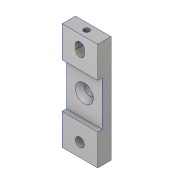
# Autodesk Inventor part: RollerBracket
Saved by Autodesk Inventor 2018 (Build 220112000, 112)
## iProperties
Created: 2020-01-17
Part Number: RollerBracket
Material: Aluminum 6061
Document SubType Name: Modeling
Designer: 22perngrac
Density: 2.7 g/cm^3
Appearance: Aluminum - Flat
Mass: 39.0791 g
Surface Area: 60.9228 cm^2
Volume: 14.4737 cm^3
Author: 22perngrac
Autodesk Inventor part; units mm, degrees
ref_plane "YZ Plane" through (0, 0, 0) normal (1, 0, 0) x (0, 1, 0)
ref_plane "XY Plane" through (0, 0, 0) normal (0, 0, 1) x (1, 0, 0)
sketch "Sketch1" plane through (0, 0, 0) normal (0, 0, 1) x (1, 0, 0)
  line L0 (0, 0) -> (25.4, 0)
  line L1 (25.4, 0) -> (25.4, 76.2)
  line L2 (25.4, 76.2) -> (0, 76.2)
  line L3 (0, 76.2) -> (0, 0)
  dimension "d0" = 76.2
  dimension "d1" = 25.4
  constraints: 8 end point, 2 parallel, 1 horizontal, 1 perpendicular
  measures "d0" distance of L0.end L1.end
  measures "d1" distance of L1.end L2.end
extrude "Extrusion1" add sketch "Sketch1" along normal blind 6.35
sketch "Sketch2" plane through (0, 0, 6.35) normal (0, 0, 1) x (1, 0, 0)
  line L0 (25.4, 76.2) -> (0, 76.2) projected
  line L1 (25.4, 0) -> (25.4, 76.2) projected
  line L2 (0, 76.2) -> (25.4, 76.2)
  line L3 (25.4, 76.2) -> (25.4, 53.975)
  line L4 (25.4, 53.975) -> (0, 53.975)
  line L5 (0, 53.975) -> (0, 76.2)
  line L6 (0, 0) -> (25.4, 0) projected
  dimension "d4" = 22.225
  constraints: 8 end point, 2 parallel, 1 horizontal, 1 perpendicular, 1 point on line
  measures "d4" distance of L4.end L0.end
extrude "Extrusion2" add sketch "Sketch2" along normal blind 3.175
ref_plane "Work Plane1" through (0, 38.1, 0) normal (0, 1, 0) x (-1, 0, 0)
mirror "Mirror1" about plane through (0, 38.1, 0) normal (0, 1, 0) of "Extrusion2"
sketch "Sketch6" plane through (0, 0, 0) normal (0, 0, 1) x (1, 0, 0)
  line L0 (25.4, 76.2) -> (0, 76.2) projected
  line L1 (25.4, 53.975) -> (25.4, 76.2) projected
  line L2 (25.4, 0) -> (0, 0) projected
  line L3 (0, 22.225) -> (25.4, 22.225) projected
  line L4 (25.4, 22.225) -> (25.4, 0) projected
  point P0 (12.7, 9.525)
  dimension "d28" = 12.7
  dimension "d29" = 12.7
  measures "d28" distance from line of point (12.7, 9.525) L3
  measures "d29" distance from line of point (12.7, 9.525) L4
sketch "Sketch7" plane through (0, 0, 6.35) normal (0, 0, 1) x (1, 0, 0)
  line L0 (0, 53.975) -> (25.4, 53.975) projected
  line L1 (0, 53.975) -> (0, 22.225) projected
  line L2 (25.4, 0) -> (25.4, 76.2) projected
  point P0 (0, 0)
  point P1 (12.7, 38.1)
  point P2 (25.4, 38.1)
  dimension "d38" = 12.7
  constraints: 1 horizontal alignment, 1 midpoint
  measures "d38" distance from line of L1 point (12.7, 38.1)
hole "Hole3" at (12.7, 38.1, 6.35) direction (0, 0, -1) diameter 6.7564 end through all countersink diameter 12.8778 countersink angle 82 clearance for "Flat Head Machine Screw (82)" size "1/4" standard "Ansi Unified Screw Threads"
hole "Hole4" at (12.7, 9.525, 0) direction (0, 0, 1) diameter 6.3754 end through all countersink diameter 12.8778 countersink angle 82 clearance for "Flat Head Machine Screw (82)" size "1/4" standard "Ansi Unified Screw Threads"
sketch "Sketch8" plane through (0, 0, 0) normal (0, 0, -1) x (-1, 0, 0)
  line L0 (-12.7, 68.2625) -> (-12.7, 65.0875) construction
  line L1 (-15.8877, 68.2625) -> (-15.8877, 65.0875)
  line L2 (-9.5123, 65.0875) -> (-9.5123, 68.2625)
  arc A0 (-9.5123, 68.2625) -> (-15.8877, 68.2625) centre (-12.7, 68.2625) ccw
  arc A1 (-15.8877, 65.0875) -> (-9.5123, 65.0875) centre (-12.7, 65.0875) ccw
  circle A2 centre (-12.7, 9.525) radius 6.4389 projected
  point P0 (-12.7, 66.675)
  point P1 (-12.7, 66.675)
  dimension "d54" = 3.175
  dimension "d67" = 57.15
  dimension "d68" = 6.3754
  constraints: 8 end point, 4 point on circle, 4 tangent, 2 centre point, 2 coincident, 1 midpoint, 1 parallel, 1 vertical
  measures "d54" distance of L1.start L1.end
  measures "d67" distance of A2.centre point (-12.7, 66.675)
  measures "d68" diameter of A0
extrude "Extrusion3" cut sketch "Sketch8" against normal through all contours A0 L2 A1 L1
sketch "Sketch10" plane through (0, 76.2, 0) normal (0, 1, 0) x (1, 0, 0)
  line L0 (0, 0) -> (0, -9.525) projected
  line L1 (25.4, 0) -> (0, 0) projected
  point P0 (12.7, -4.7625)
  point P1 (0, -4.7625)
  point P2 (12.7, 0)
  constraints: 2 midpoint, 1 horizontal alignment, 1 vertical alignment
hole "Hole5" at (12.7, 76.2, 4.7625) direction (0, -1, 0) diameter 3.9624 depth 9.525 tip angle 118 thread size "10-32 UNF" class "2B" standard "ANSI Unified Screw Threads"
body "Solid1"
